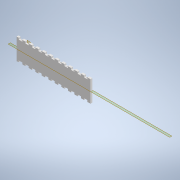
# Autodesk Inventor part: 00_Baseplate_Simmo_side3
Saved by Autodesk Inventor 2022 (Build 260153000, 153)
## iProperties
Created: 2022-04-28
Part Number: 00_Baseplate_Simmo_side3
Material: Generisch
Document SubType Name: Modeling
Designer: diederichbenedict
Density: 1 g/cm^3
Appearance: Vorgabe
Author: diederichbenedict
Autodesk Inventor part; units mm, degrees
ref_plane "YZ Plane" through (0, 0, 0) normal (1, 0, 0) x (0, 1, 0)
ref_plane "XZ Plane" through (0, 0, 0) normal (0, 1, 0) x (-1, 0, 0)
ref_plane "XY Plane" through (0, 0, 0) normal (0, 0, 1) x (1, 0, 0)
ref_plane "Arbeitsebene1" through (0, 0, 0) normal (0, 0, 1) x (1, 0, 0)
sketch "Skizze1" plane through (0, 0, 0) normal (0, 0, 1) x (1, 0, 0)
  line L0 (0, 20) -> (229.5237, 20)
  line L1 (229.5237, 20) -> (229.5237, -54)
  line L2 (229.5237, -54) -> (0, -54)
  line L3 (0, -54) -> (0, 20)
  line L4 (0, -54) -> (229.5237, -54)
  line L5 (229.5237, -54) -> (229.5237, -60)
  line L6 (229.5237, -60) -> (0, -60)
  line L7 (0, -60) -> (0, -54)
  line L8 (2.7577, 20) -> (-3.0026, 20) projected
  point P0 (450, -68)
  point P1 (450, -68)
  dimension "d0" = 6
  constraints: 16 end point, 4 parallel, 2 horizontal, 2 perpendicular, 1 point on line
  measures "d0" distance of L1.end L5.end
extrude "Extrusion1" add sketch "Skizze1" along normal blind 6
sketch "Skizze2" plane through (0, 0, 0) normal (0, 0, -1) x (1, 0, 0)
  line L0 (0, -20) -> (0, 60) projected
  line L1 (9.8, -20) -> (20.2, -20)
  line L2 (20.2, -20) -> (20.2, -14)
  line L3 (20.2, -14) -> (9.8, -14)
  line L4 (9.8, -14) -> (9.8, -20)
  point P0 (0, 0)
  dimension "d38" = 0
  dimension "d39" = 6
  constraints: 8 end point, 2 parallel, 1 horizontal, 1 perpendicular
  measures "d38" vertical distance of L1.start L0.start
  measures "d39" distance between parallel lines of L3 L1
extrude "Extrusion2" cut sketch "Skizze2" against normal blind 6
sketch "Skizze3" plane through (20.2, 20, 0) normal (0, 1, 0) x (1, 0, 0)
  line L0 (209.3237, 0) -> (0, 0) projected
  line L1 (-10.4, -6) -> (0, -6) projected
  line L2 (0, 0) -> (0, -6) projected
  circle A0 centre (-5.2, -3) radius 1.5
  line L3 (-10.4, -6) -> (-10.4, 0) projected
  point P0 (-20.2, 0)
  point P1 (4.8, 3)
  point P2 (429.8, 0)
  point P3 (429.8, -6)
  dimension "d16" = 3
  dimension "d19" = 5.2
  constraints: 1 centre point
  measures "d16" diameter of A0
  measures "d19" distance from line of A0.centre L3
hole "Bohrung1" at (15, 20, 3) direction (0, -1, 0) diameter 3 depth 20
pattern_linear "Rechteckige Anordnung1" count 24 spacing 20 along (1, 0, 0) of "Extrusion2", "Bohrung1"
ref_plane "Arbeitsebene2" through (20.2, -20, 6) normal (0, 1, 0) x (1, 0, 0)
mirror "Spiegeln1" about plane through (20.2, -20, 6) normal (0, 1, 0) of "Extrusion2", "Bohrung1", "Rechteckige Anordnung1"
sketch "Skizze4" plane through (0, 5, 6) normal (0, 1, 0) x (1, 0, 0)
  line L0 (9.8356, 19.8689) -> (14.6897, 16.3421) projected
  line L1 (20.45, 24.2705) -> (14.6897, 16.3421) projected
  line L2 (15.5959, 27.7972) -> (20.45, 24.2705) projected
  line L3 (15.5959, 27.7972) -> (9.8356, 19.8689) projected
  line L4 (9.8, 0) -> (0, 0) projected
  line L5 (3, 0) -> (-2.0103, 0)
  line L6 (-2.0103, 0) -> (-2.0103, 6)
  line L7 (-2.0103, 6) -> (3, 6)
  line L8 (3, 6) -> (3, 0)
  line L9 (0, 6) -> (0, 0) projected
  line L10 (2.8165, 0) -> (2.8165, 6)
  point P0 (-2.0103, 2.2794)
  point P1 (0, 6)
  point P2 (0, 0)
  point P3 (0, 0)
  dimension "d25" = 3
  constraints: 10 end point, 2 parallel, 1 horizontal, 1 perpendicular, 1 point on line, 1 vertical, 3 other
  measures "d25" distance between parallel lines of L9 L8
extrude "Extrusion3" [suppressed]
